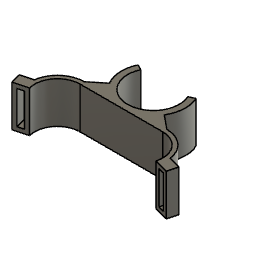
battery_mount (Autodesk Fusion 360 design; units mm, degrees)
Autodesk Fusion 360 part; units mm, degrees
sketch "Sketch1" plane through (0, 0, 0) normal (0, 1, 0) x (1, 0, 0)
  circle A0 centre (0, 0) radius 12.5
  circle A1 centre (0, 0) radius 15.5
  line L0 (0, 0) -> (14.0478, 6.5506)
  line L1 (0, 0) -> (15.5, 0) construction
  line L2 (0, 0) -> (-14.3059, 6.671)
  line L3 (0, -15) -> (0, -15.5)
  line L4 (0, -15.5) -> (31, -15.5)
  line L5 (31, -15.5) -> (-31, -15.5)
  circle A2 centre (20, -26.5) radius 11
  circle A3 centre (-20, -26.5) radius 11
  circle A4 centre (-20, -26.5) radius 13
  circle A5 centre (20, -26.5) radius 13
  line L6 (-20, -26.5) -> (-32.557, -29.8646)
  line L7 (-20, -26.5) -> (-7, -26.5) construction
  line L8 (20, -26.5) -> (32.557, -29.8646)
  line L9 (20, -26.5) -> (33, -26.5) construction
  line L10 (-20, -14) -> (-20, -13.5)
  line L11 (20, -14) -> (20, -13.5)
  line L12 (-20, -13.5) -> (-13.2759, -8)
  line L13 (13.2759, -8) -> (20, -13.5)
  line L14 (-32.557, -29.8646) -> (-33.8511, -25.035)
  line L15 (-33.8511, -25.035) -> (-38.6808, -26.3291)
  line L16 (-38.6808, -26.3291) -> (-37.3867, -31.1587)
  line L17 (-37.3867, -31.1587) -> (-32.557, -29.8646)
  line L18 (-33.8511, -25.035) -> (-32.8852, -24.7762)
  line L19 (32.557, -29.8646) -> (33.8511, -25.035)
  line L20 (33.8511, -25.035) -> (38.6808, -26.3291)
  line L21 (38.6808, -26.3291) -> (37.3867, -31.1587)
  line L22 (37.3867, -31.1587) -> (32.557, -29.8646)
  line L23 (33.8511, -25.035) -> (32.8852, -24.7762)
  dimension "d1" = 25
  dimension "d2" = 31
  dimension "d3" = 25
  dimension "d4" = 50
  dimension "d5" = 31
  dimension "d6" = 62
  dimension "d8" = 26
  dimension "d9" = 26
  dimension "d10" = 165
  dimension "d11" = 15
  dimension "d12" = 5
  dimension "d13" = 5
  dimension "d14" = 5
  constraint coincident A0.centre A1.centre
  constraint horizontal L1
  constraint coincident A1 L3.end
  constraint vertical L3
  constraint perpendicular L3 L4
  constraint horizontal L5
  constraint tangent L5 A2
  constraint tangent L5 A3
  constraint concentric A3 A4
  constraint concentric A2 A5
  constraint horizontal L7
  constraint coincident A3.centre A4.centre
  constraint horizontal L9
  constraint coincident A2.centre A5.centre
  constraint coincident A4 L10.end
  constraint perpendicular L5 L10
  constraint coincident A5 L11.end
  constraint perpendicular L5 L11
  constraint coincident A1 L13.start
  constraint coincident A1 L12.end
  constraint perpendicular L14 L15
  constraint parallel L14 L16
  constraint parallel L15 L17
  constraint perpendicular L6 L14
  constraint coincident A4 L18.end
  constraint perpendicular L14 L18
  constraint perpendicular L19 L20
  constraint parallel L19 L21
  constraint parallel L20 L22
  constraint tangent A5 L19
  constraint perpendicular L8 L19
  constraint coincident A5 L23.end
  constraint perpendicular L19 L23
  measures "d1" diameter of A0
  measures "d2" diameter of A1
  measures "d3" angle of L0 L1
  measures "d4" angle of L0 L2
  measures "d5" distance of L3.end L4.end
  measures "d6" distance of L4.end L5.end
  measures "d8" diameter of A4
  measures "d9" diameter of A5
  measures "d10" angle of L6 L7
  measures "d11" angle of L8 L9
  measures "d12" distance of L6.end L16.end
  measures "d13" distance of L8.end L19.end
  measures "d14" distance of L8.end L21.end
extrude "Extrude1" add sketch "Sketch1" along normal blind 20 contours A0 A1 L0 L2 | A1 L5 A4 L12 | A1 L4 L5 A5 L13 | L5 A4 | L4 L5 A5 | L5 A3 A4 L6 | L4 L5 A2 A5 L8 | A5 L19 L23 | L19 L20 L21 L22 | A4 L14 L18 | L14 L15 L16 L17 picked at (-5.1968, -13.5069) picked at (-32.0801, -24.1441) picked at (32.0902, -24.2104)
sketch "Sketch2" plane through (5.2853, 0, 19.7248) normal (0.258819, 0, 0.965926) x (0.965926, 0, -0.258819)
  line L0 (-44.1772, 0) -> (-37.1772, 0)
  line L1 (-37.1772, 0) -> (-37.1772, 20)
  line L2 (-37.1772, 20) -> (-44.1772, 20)
  line L3 (-44.1772, 20) -> (-44.1772, 0)
  line L4 (-44.1772, 20) -> (-42.1772, 20)
  line L5 (-42.1772, 20) -> (-42.1772, 2)
  line L6 (-42.1772, 2) -> (-44.1772, 2)
  line L7 (-44.1772, 2) -> (-44.1772, 20)
  line L8 (-42.1772, 2) -> (-39.1772, 2)
  line L9 (-39.1772, 2) -> (-39.1772, 18)
  line L10 (-39.1772, 18) -> (-42.1772, 18)
  line L11 (-42.1772, 18) -> (-42.1772, 2)
  dimension "d17" = 2
  dimension "d18" = 18
  dimension "d19" = 3
  dimension "d20" = 16
  constraint horizontal L4
  constraint vertical L5
  constraint horizontal L6
  constraint vertical L7
  constraint coincident L2.end L3.start
  constraint horizontal L8
  constraint vertical L9
  constraint horizontal L10
  constraint vertical L11
  measures "d17" distance of L2.end L4.end
  measures "d18" distance of L2.end L6.end
  measures "d19" distance of L5.end L8.end
  measures "d20" distance of L5.end L10.end
extrude "Extrude2" cut sketch "Sketch2" against normal blind 5 contours L5 L8 L9 L10 L11
sketch "Sketch3" plane through (-5.2853, 0, 19.7248) normal (-0.258819, 0, 0.965926) x (0.965926, 0, 0.258819)
  line L0 (37.1772, 0) -> (44.1772, 0)
  line L1 (44.1772, 0) -> (44.1772, 20)
  line L2 (44.1772, 20) -> (37.1772, 20)
  line L3 (37.1772, 20) -> (37.1772, 0)
  line L4 (44.1772, 20) -> (42.1772, 20)
  line L5 (42.1772, 20) -> (42.1772, 2)
  line L6 (42.1772, 2) -> (44.1772, 2)
  line L7 (44.1772, 2) -> (44.1772, 20)
  line L8 (42.1772, 2) -> (39.1772, 2)
  line L9 (39.1772, 2) -> (39.1772, 18)
  line L10 (39.1772, 18) -> (42.1772, 18)
  line L11 (42.1772, 18) -> (42.1772, 2)
  dimension "d23" = 2
  dimension "d24" = 18
  dimension "d25" = 3
  dimension "d26" = 16
  constraint horizontal L4
  constraint vertical L5
  constraint horizontal L6
  constraint vertical L7
  constraint coincident L1.end L2.start
  constraint vertical L9
  constraint perpendicular L8 L9
  constraint horizontal L10
  constraint vertical L11
  measures "d23" distance of L1.end L4.end
  measures "d24" distance of L1.end L6.end
  measures "d25" distance of L5.end L8.end
  measures "d26" distance of L5.end L10.end
extrude "Extrude3" cut sketch "Sketch3" against normal blind 6 contours L5 L8 L9 L10 L11
equation "d4 = d3 * 2"
equation "d6 = d5 * 2"
